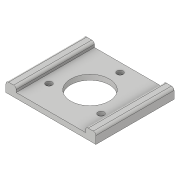
# Autodesk Inventor part: soporte inferior ridgid -2
Saved by Autodesk Inventor 2019 (Build 230136000, 136)
## iProperties
Created: 2019-11-12
Part Number: soporte inferior ridgid -2
Material: Generic
Document SubType Name: Modeling
Designer: Carlos Andres garcia velez
Density: 1 g/cm^3
Appearance: Default
Author: Carlos Andres garcia velez
Autodesk Inventor part; units mm, degrees
ref_plane "YZ Plane" through (0, 0, 0) normal (1, 0, 0) x (0, 1, 0)
ref_plane "XZ Plane" through (0, 0, 0) normal (0, 1, 0) x (-1, 0, 0)
ref_plane "XY Plane" through (0, 0, 0) normal (0, 0, 1) x (1, 0, 0)
sketch "Sketch1" plane through (0, 0, 0) normal (0, 1, 0) x (-1, 0, 0)
  line L0 (-30.1299, 69.45) -> (30.245, 69.45)
  line L1 (30.245, -69.45) -> (-30.1299, -69.45)
  circle A0 centre (0, 0) radius 37.5
  arc A1 (-30.1299, 69.45) -> (-30.1299, -69.45) centre (0, 0) ccw
  arc A2 (30.245, -69.45) -> (30.245, 69.45) centre (0, 0) ccw
  circle A3 centre (0, -58.5) radius 6
  circle A4 centre (0, -58.5) radius 3.25
  circle A5 centre (0, 0) radius 45.75 construction
  circle A6 centre (50.6625, 29.25) radius 6
  circle A7 centre (50.6625, 29.25) radius 3.25
  circle A8 centre (-50.6625, 29.25) radius 6
  circle A9 centre (-50.6625, 29.25) radius 3.25
  line L2 (87.5, -76) -> (-87.5, -76)
  line L3 (-87.5, -76) -> (-87.5, 76)
  line L4 (-87.5, 76) -> (87.5, 76)
  line L5 (87.5, 76) -> (87.5, -76)
  point P0 (-87.5, 0)
  point P1 (0, -76)
  dimension "d1" = 75
  dimension "d2" = 69.45
  dimension "d3" = 58.5
  dimension "d4" = 12
  dimension "d5" = 6.5
  dimension "d8" = 360
  dimension "d57" = 75.75
  dimension "d58" = 69.45
  dimension "d59" = 69.45
  dimension "d69" = 152
  dimension "d70" = 175
  constraints: 12 end point, 10 centre point, 5 coincident, 4 point on circle, 3 parallel, 2 horizontal, 2 midpoint, 1 horizontal alignment, 1 perpendicular, 1 vertical alignment, 13 other
  measures "d1" diameter of A0
  measures "d2" distance from line of L1 A0.centre
  measures "d3" distance of A0.centre A3.centre
  measures "d4" diameter of A3
  measures "d5" diameter of A4
  measures "d57" radius of A2
  measures "d58" distance from line of point (0, 0) L0
  measures "d59" distance from line of point (0, 0) L1
  measures "d69" distance of L2.end L3.end
  measures "d70" distance of L2.start L2.end
extrude "Extrusion1" add sketch "Sketch1" along normal blind 10 contours L0 A2 L1 A1 | A3 | A6 | A8 | L2 L3 L4 L5
sketch "Sketch2" plane through (0, 10, 0) normal (0, 1, 0) x (1, 0, 0)
  circle A0 centre (0, 58.5) radius 3.25 projected
  circle A1 centre (0, 58.5) radius 6
  circle A2 centre (50.6625, -29.25) radius 3.25 projected
  circle A3 centre (50.6625, -29.25) radius 6
  circle A4 centre (-50.6625, -29.25) radius 3.25 projected
  circle A5 centre (-50.6625, -29.25) radius 6
  point P0 (0, 0)
  dimension "d12" = 12
  dimension "d13" = 12
  dimension "d14" = 12
  constraints: 3 centre point, 3 coincident
  measures "d12" diameter of A1
  measures "d13" diameter of A3
  measures "d14" diameter of A5
extrude "Extrusion2" cut sketch "Sketch2" against normal blind 6.5
sketch "Sketch11" plane through (0, 10, 0) normal (0, 1, 0) x (1, 0, 0)
  circle A0 centre (-50.6625, -29.25) radius 6 projected
  circle A1 centre (0, 58.5) radius 6 projected
  circle A2 centre (50.6625, -29.25) radius 6 projected
  circle A3 centre (0, 0) radius 37.5 projected
  line L0 (87.5, 76) -> (-87.5, 76) projected
  line L1 (-87.5, 76) -> (-87.5, -76) projected
  line L2 (-87.5, -76) -> (87.5, -76) projected
  line L3 (87.5, -76) -> (87.5, 76) projected
  line L4 (-87.5, 76) -> (-67.5, 76)
  line L5 (-67.5, 76) -> (-67.5, -76)
  line L6 (-67.5, -76) -> (-87.5, -76)
  line L7 (-87.5, -76) -> (-87.5, 76)
  line L8 (87.5, 76) -> (-87.5, 76) projected
  line L9 (87.5, -76) -> (-87.5, -76) projected
  line L10 (87.5, 76) -> (67.5, 76)
  line L11 (67.5, 76) -> (67.5, -76)
  line L12 (67.5, -76) -> (87.5, -76)
  line L13 (87.5, -76) -> (87.5, 76)
  point P0 (0, 0)
  dimension "d71" = 20
  dimension "d72" = 20
  constraints: 16 end point, 4 parallel, 2 horizontal, 2 perpendicular, 2 point on line
  measures "d71" distance of L5.end L6.end
  measures "d72" distance of L12.end L11.end
extrude "Extrusion11" add sketch "Sketch11" along normal blind 10 contours L3 L2 L11 L0 | L5 L2 L1 L0
fillet "Fillet9" radius 5 4 edges at (-67.5, 20, 0) (-87.5, 20, 0) (67.5, 20, 0) (87.5, 20, 0)
equation "\"d2\" = d59"
equation "\"d59\" = d58"
body "Solid1"
